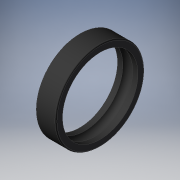
# Autodesk Inventor part: 60/28 Outer Ring
Saved by Autodesk Inventor 2019 (Build 230136000, 136)
## iProperties
Created: 2024-02-20
Part Number: 60/28 Outer Ring
Material: Generic
Catalog Web Link: www.cadenas.de
Description: Open type or-Deep Groove Ball Bearings
Vendor: NTN
Document SubType Name: Modeling
Designer: psAdmin
Manufacturer: NTN
Mass: 6.11822 g
Surface Area: 48.7599 cm^2
Volume: 6.11822 cm^3
Density: 1 g/cm^3
Appearance: PSOLRGB-175-175-175
Category: PARTsolutions
Company: NTN
Title: 60/28 Outer Ring
Author: Cadenas PARTsolutions
Comments: Deep Groove Ball Bearings
PSOL_IDENT_0: {$CADENAS_DATA/23d-libs/ntn/ball_roller_bearings/deep_groove_bb/deep_groove_bb/6_types/dgbb_or.prj},
PSOL_IDENT_1: 179 {VTYP=3D},{NB=60/28 Outer Ring},{LINA=60/28 Outer Ring},{NN=Open type or},{DATE=17.10.2023 22:55
PSOL_IDENT_2: :17},{GEOMDATE=13.03.2020 06:48:21},{VERSION=},{LINEID=480},{WBVAR=},{WBNUMERIC=}  {NB=60/28 Outer R
PSOL_IDENT_3: ing},{LINA=60/28 Outer Ring},{KT=DUMMY},{IDNR=},{SD=28},{D=52},{B=12},{R=0.6},{ORDER1=60/28},{ORDER=
PSOL_IDENT_4: 60/28},{NEWORDER=60/28},{CR=12.5},{COR=7.40},{CRF=1270},{CORF=755},{LSG=14000},{LSO=16000},{MASS=0.1
PSOL_IDENT_5: 0},{RNS=0.5},{LLH=10000},{LLU=8400},{ST=ZZ},{NCST=LLB},{LTST=LLH},{CST=LLU},{SRG=N},{SR=NR},{D1=49.7
PSOL_IDENT_6: 3},{A=2.06},{BA=1.35},{R0=0.40},{D2=57.9},{F=1.12},{DA1=32},{DA2=34},{DA=48},{DX=58.5},{CY=2.9},{CZ=
PSOL_IDENT_7: 1.2},{RAS=0.6},{RNAS=0.5},{VERS=1},{X=12},{N=10},{RB=3.60000},{O=125.60000}
NB: 60/28 Outer Ring
NN: Open type or
NT: Deep Groove Ball Bearings
NBSYN: $ORDER. Outer Ring
LINA: 60/28 Outer Ring
CATALOG: NTN Corporation
SD: 28
D: 52
B: 12
R: 0.6
ORDER1: 60/28
ORDER: 60/28
NEWORDER: 60/28
CR: 12.5
COR: 7.40
CRF: 1270
CORF: 755
LSG: 14000
LSO: 16000
MASS: 0.10
RNS: 0.5
LLH: 10000
LLU: 8400
ST: ZZ
NCST: LLB
LTST: LLH
CST: LLU
SRG: N
SR: NR
D1: 49.73
A: 2.06
BA: 1.35
R0: 0.4
D2: 57.9
F: 1.12
DA1: 32
DA2: 34
DA: 48
DX: 58.5
CY: 2.9
CZ: 1.2
RAS: 0.6
RNAS: 0.5
VERS: 1
SUPPLIER: NTN
ARTICLENO: 60/28 Outer Ring
BOMINFO: 60/28 Outer Ring
CREATOR: CADENAS GmbH
Autodesk Inventor part; units mm, degrees
sketch "Sketch_1" plane through (0, 0, 0) normal (0, 0, 1) x (1, 0, 0)
  line L0 (12, 0) -> (0, 0)
  line L1 (0, 22.16) -> (3.12, 22.16)
  arc A0 (8.88, 22.16) -> (3.12, 22.16) centre (6, 20) ccw
  line L2 (8.88, 22.16) -> (12, 22.16)
  line L3 (12, 22.16) -> (12, 25.4)
  arc A1 (12, 25.4) -> (11.4, 26) centre (11.4, 25.4) ccw
  line L4 (11.4, 26) -> (0.6, 26)
  arc A2 (0.6, 26) -> (0, 25.4) centre (0.6, 25.4) ccw
  line L5 (0, 25.4) -> (0, 22.16)
  constraints: 12 end point, 6 point on circle, 3 centre point
revolve "Revolution1" add sketch "Sketch_1" angle 360 about axis through (12, 0, 0) along (1, 0, 0)
ref_plane "dgbb_or_XY" through (0, 0, 0) normal (1, 0, 0) x (0, 0, -1)
ref_plane "dgbb_or_YZ" through (0, 0, 0) normal (0, 0, -1) x (0, 1, 0)
ref_plane "dgbb_or_ZX" through (0, 0, 0) normal (0, 1, 0) x (1, 0, 0)
ref_plane "dgbb_or1_XY" through (12, 0, 0) normal (1, 0, 0) x (0, 0, -1)
ref_plane "dgbb_or1_YZ" through (12, 0, 0) normal (0, 0, -1) x (0, 1, 0)
ref_plane "dgbb_or1_ZX" through (12, 0, 0) normal (0, 1, 0) x (1, 0, 0)
ref_plane "dgbb_or11_1_XY" through (6, 20, 0) normal (1, 0, 0) x (0, 0, -1)
ref_plane "dgbb_or11_1_YZ" through (6, 20, 0) normal (0, 0, -1) x (0, 1, 0)
ref_plane "dgbb_or11_1_ZX" through (6, 20, 0) normal (0, 1, 0) x (1, 0, 0)
ref_plane "dgbb_or11_10_XY" through (6, 16.1803, -11.7557) normal (1, 0, 0) x (0, 0, -1)
ref_plane "dgbb_or11_10_YZ" through (6, 16.1803, -11.7557) normal (0, 0, -1) x (0, 1, 0)
ref_plane "dgbb_or11_10_ZX" through (6, 16.1803, -11.7557) normal (0, 1, 0) x (1, 0, 0)
ref_plane "dgbb_or11_2_XY" through (6, 16.1803, 11.7557) normal (1, 0, 0) x (0, 0, -1)
ref_plane "dgbb_or11_2_YZ" through (6, 16.1803, 11.7557) normal (0, 0, -1) x (0, 1, 0)
ref_plane "dgbb_or11_2_ZX" through (6, 16.1803, 11.7557) normal (0, 1, 0) x (1, 0, 0)
ref_plane "dgbb_or11_3_XY" through (6, 6.1803, 19.0211) normal (1, 0, 0) x (0, 0, -1)
ref_plane "dgbb_or11_3_YZ" through (6, 6.1803, 19.0211) normal (0, 0, -1) x (0, 1, 0)
ref_plane "dgbb_or11_3_ZX" through (6, 6.1803, 19.0211) normal (0, 1, 0) x (1, 0, 0)
ref_plane "dgbb_or11_4_XY" through (6, -6.1803, 19.0211) normal (1, 0, 0) x (0, 0, -1)
ref_plane "dgbb_or11_4_YZ" through (6, -6.1803, 19.0211) normal (0, 0, -1) x (0, 1, 0)
ref_plane "dgbb_or11_4_ZX" through (6, -6.1803, 19.0211) normal (0, 1, 0) x (1, 0, 0)
ref_plane "dgbb_or11_5_XY" through (6, -16.1803, 11.7557) normal (1, 0, 0) x (0, 0, -1)
ref_plane "dgbb_or11_5_YZ" through (6, -16.1803, 11.7557) normal (0, 0, -1) x (0, 1, 0)
ref_plane "dgbb_or11_5_ZX" through (6, -16.1803, 11.7557) normal (0, 1, 0) x (1, 0, 0)
ref_plane "dgbb_or11_6_XY" through (6, -20, 0) normal (1, 0, 0) x (0, 0, -1)
ref_plane "dgbb_or11_6_YZ" through (6, -20, 0) normal (0, 0, -1) x (0, 1, 0)
ref_plane "dgbb_or11_6_ZX" through (6, -20, 0) normal (0, 1, 0) x (1, 0, 0)
ref_plane "dgbb_or11_7_XY" through (6, -16.1803, -11.7557) normal (1, 0, 0) x (0, 0, -1)
ref_plane "dgbb_or11_7_YZ" through (6, -16.1803, -11.7557) normal (0, 0, -1) x (0, 1, 0)
ref_plane "dgbb_or11_7_ZX" through (6, -16.1803, -11.7557) normal (0, 1, 0) x (1, 0, 0)
ref_plane "dgbb_or11_8_XY" through (6, -6.1803, -19.0211) normal (1, 0, 0) x (0, 0, -1)
ref_plane "dgbb_or11_8_YZ" through (6, -6.1803, -19.0211) normal (0, 0, -1) x (0, 1, 0)
ref_plane "dgbb_or11_8_ZX" through (6, -6.1803, -19.0211) normal (0, 1, 0) x (1, 0, 0)
ref_plane "dgbb_or11_9_XY" through (6, 6.1803, -19.0211) normal (1, 0, 0) x (0, 0, -1)
ref_plane "dgbb_or11_9_YZ" through (6, 6.1803, -19.0211) normal (0, 0, -1) x (0, 1, 0)
ref_plane "dgbb_or11_9_ZX" through (6, 6.1803, -19.0211) normal (0, 1, 0) x (1, 0, 0)
body "Solid1"
